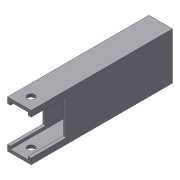
# Autodesk Inventor part: Frame_LowerRollerMount
Saved by Autodesk Inventor 2012 (Build 160160000, 160)
## iProperties
Created: 2012-01-14
Part Number: Frame_LowerRollerMount
Material: Aluminum-6061
Document SubType Name: Modeling
Designer: JesseK
Density: 2.71 g/cm^3
Mass: 157.355 g
Surface Area: 381.055 cm^2
Volume: 58.0647 cm^3
Author: JesseK
Autodesk Inventor part; units mm, degrees
ref_plane "YZ Plane" through (0, 0, 0) normal (1, 0, 0) x (0, 1, 0)
ref_plane "XZ Plane" through (0, 0, 0) normal (0, 1, 0) x (-1, 0, 0)
ref_plane "XY Plane" through (0, 0, 0) normal (0, 0, 1) x (1, 0, 0)
sketch "Sketch1" plane through (0, 0, 0) normal (0, 0, 1) x (1, 0, 0)
  line L0 (0, 0) -> (25.4, 0)
  line L1 (25.4, 0) -> (25.4, 50.8)
  line L2 (25.4, 50.8) -> (0, 50.8)
  line L3 (0, 50.8) -> (0, 0)
  dimension "d0" = 25.4
  dimension "d1" = 50.8
  constraints: 8 end point, 2 parallel, 1 horizontal, 1 perpendicular
  measures "d0" distance of L1.end L2.end
  measures "d1" distance of L2.end L0.start
extrude "Extrusion1" add sketch "Sketch1" along normal blind 152.4
shell "Shell1" thickness 3.175 removed faces 2 at (8.4667, 33.8667, 0) at (8.4667, 33.8667, 152.4)
sketch "Sketch4" plane through (25.4, 0, 0) normal (1, 0, 0) x (0, 0, -1)
  line L0 (-152.4, 50.8) -> (-152.4, 0) projected
  line L1 (0, 0) -> (-152.4, 0) projected
  line L2 (0, 50.8) -> (-152.4, 50.8) projected
  line L3 (-152.4, 44.45) -> (-114.3, 44.45)
  line L4 (-114.3, 44.45) -> (-114.3, 6.35)
  line L5 (-114.3, 6.35) -> (-152.4, 6.35)
  line L6 (-152.4, 6.35) -> (-152.4, 44.45)
  dimension "d15" = 6.35
  dimension "d16" = 6.35
  dimension "d17" = 38.1
  constraints: 8 end point, 2 parallel, 1 horizontal, 1 perpendicular, 1 point on line
  measures "d15" distance between parallel lines of L2 L3
  measures "d16" distance between parallel lines of L1 L5
  measures "d17" distance of L4.end L5.end
extrude "Extrusion4" cut sketch "Sketch4" against normal through all
sketch "Sketch5" plane through (0, 50.8, 0) normal (0, 1, 0) x (1, 0, 0)
  line L0 (0, -152.4) -> (25.4, -152.4) projected
  line L1 (25.4, 0) -> (25.4, -152.4) projected
  circle A0 centre (12.7, -139.7) radius 3.9688
  dimension "d20" = 7.9375
  dimension "d21" = 12.7
  dimension "d22" = 12.7
  constraints: 1 centre point
  measures "d20" diameter of A0
  measures "d21" distance from line of L0 A0.centre
  measures "d22" distance from line of L1 A0.centre
extrude "Extrusion5" cut sketch "Sketch5" against normal through all
body "Solid1"
